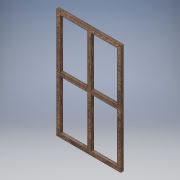
# Autodesk Inventor part: Door
Saved by Autodesk Inventor 2017 (Build 210142000, 142)
## iProperties
Created: 2016-09-12
Part Number: Door
Material: Generic
Document SubType Name: Modeling
Designer: s.ethan.wierenga
Density: 1 g/cm^3
Appearance: White Ash - Java
Author: s.ethan.wierenga
Autodesk Inventor part; units mm, degrees
ref_plane "YZ Plane" through (0, 0, 0) normal (1, 0, 0) x (0, 1, 0)
ref_plane "XZ Plane" through (0, 0, 0) normal (0, 1, 0) x (-1, 0, 0)
ref_plane "XY Plane" through (0, 0, 0) normal (0, 0, 1) x (1, 0, 0)
sketch "Sketch1" plane through (0, 0, 0) normal (0, 0, 1) x (1, 0, 0)
  line L0 (0, 0) -> (457.2, 0)
  line L1 (457.2, 0) -> (457.2, 781.05)
  line L2 (457.2, 781.05) -> (0, 781.05)
  line L3 (0, 781.05) -> (0, 0)
  dimension "d0" = 457.2
  dimension "d1" = 781.05
  constraints: 8 end point, 2 parallel, 1 horizontal, 1 perpendicular
  measures "d0" distance of L2.end L1.end
  measures "d1" distance of L0.end L1.end
extrude "Extrusion1" add sketch "Sketch1" along normal blind 19.05
sketch "Sketch2" plane through (0, 0, 19.05) normal (0, 0, 1) x (1, 0, 0)
  line L0 (0, 0) -> (457.2, 0) projected
  line L1 (457.2, 0) -> (457.2, 781.05) projected
  line L2 (457.2, 781.05) -> (0, 781.05) projected
  line L3 (0, 781.05) -> (0, 0) projected
  line L4 (25.4, 755.65) -> (220.6625, 755.65)
  line L5 (220.6625, 755.65) -> (220.6625, 403.225)
  line L6 (220.6625, 403.225) -> (25.4, 403.225)
  line L7 (25.4, 403.225) -> (25.4, 755.65)
  line L8 (246.0625, 755.65) -> (431.8, 755.65)
  line L9 (431.8, 755.65) -> (431.8, 403.225)
  line L10 (431.8, 403.225) -> (246.0625, 403.225)
  line L11 (246.0625, 403.225) -> (246.0625, 755.65)
  line L12 (25.4, 377.825) -> (220.6625, 377.825)
  line L13 (220.6625, 377.825) -> (220.6625, 25.4)
  line L14 (220.6625, 25.4) -> (25.4, 25.4)
  line L15 (25.4, 25.4) -> (25.4, 377.825)
  line L16 (246.0625, 377.825) -> (431.8, 377.825)
  line L17 (431.8, 377.825) -> (431.8, 25.4)
  line L18 (431.8, 25.4) -> (246.0625, 25.4)
  line L19 (246.0625, 25.4) -> (246.0625, 377.825)
  dimension "d24" = 25.4
  dimension "d25" = 25.4
  dimension "d26" = 25.4
  dimension "d27" = 25.4
  dimension "d28" = 25.4
  dimension "d29" = 25.4
  dimension "d30" = 25.4
  dimension "d31" = 25.4
  dimension "d32" = 25.4
  dimension "d33" = 25.4
  dimension "d34" = 185.7375
  dimension "d35" = 195.2625
  dimension "d36" = 352.425
  constraints: 32 end point, 8 parallel, 4 horizontal, 4 perpendicular, 4 point on line
  measures "d24" distance between parallel lines of L2 L4
  measures "d25" distance between parallel lines of L0 L14
  measures "d26" distance between parallel lines of L3 L15
  measures "d27" distance between parallel lines of L3 L7
  measures "d28" distance between parallel lines of L1 L9
  measures "d29" distance between parallel lines of L1 L17
  measures "d30" distance between parallel lines of L10 L16
  measures "d31" distance between parallel lines of L6 L12
  measures "d32" distance between parallel lines of L11 L5
  measures "d33" distance between parallel lines of L19 L13
  measures "d34" distance of L16.start L16.end
  measures "d35" distance of L5.end L6.end
  measures "d36" distance of L8.end L9.end
extrude "Extrusion2" cut sketch "Sketch2" against normal blind 19.05 contours L4 L5 L6 L7 | L8 L9 L10 L11 | L12 L13 L14 L15 | L16 L17 L18 L19
body "Solid1"
